Autodesk Fusion 360 part; units mm, degrees
(part 2 of 2)
  spline S109 degree 3 poles (28.856, 5.5784) (28.9294, 5.4954) (29.0682, 5.3385) (29.2744, 5.3081) (29.3716, 5.2937) knots 0 0 0 0 0.032048 0.06061 0.06061 0.06061 0.06061
  spline S110 degree 3 poles (29.3716, 5.2937) (29.4328, 5.2987) (29.5558, 5.3088) (29.6585, 5.3774) (29.71, 5.4119) knots 0 0 0 0 0.018102 0.036374 0.036374 0.036374 0.036374
  spline S111 degree 3 poles (29.71, 5.4119) (29.7609, 5.46) (29.8723, 5.5653) (29.9342, 5.706) (29.9678, 5.7825) knots 0 0 0 0 0.020804 0.045551 0.045551 0.045551 0.045551
  spline S112 degree 3 poles (29.9678, 5.7825) (29.9978, 5.8777) (30.0869, 6.1604) (30.1638, 6.4466) (30.2149, 6.6365) knots 0 0 0 0 0.029943 0.088911 0.088911 0.088911 0.088911
  spline S113 degree 3 poles (30.2149, 6.6365) (30.2924, 6.9284) (30.4207, 7.4117) (30.5964, 7.8798) (30.6661, 8.0652) knots 0 0 0 0 0.090525 0.149905 0.149905 0.149905 0.149905
  spline S114 degree 3 poles (30.6661, 8.0652) (30.7287, 8.1929) (30.8511, 8.4425) (31.066, 8.6184) (31.1709, 8.7043) knots 0 0 0 0 0.042122 0.082304 0.082304 0.082304 0.082304
  spline S115 degree 3 poles (31.1709, 8.7043) (31.2926, 8.7716) (31.5496, 8.9138) (31.8434, 8.9279) (31.9981, 8.9353) knots 0 0 0 0 0.041152 0.086904 0.086904 0.086904 0.086904
  spline S116 degree 3 poles (31.9981, 8.9353) (32.1582, 8.9226) (32.4839, 8.8969) (32.7671, 8.7336) (32.9112, 8.6506) knots 0 0 0 0 0.047533 0.09672 0.09672 0.09672 0.09672
  spline S117 degree 3 poles (32.9112, 8.6506) (33.0461, 8.544) (33.326, 8.3228) (33.4879, 8.0045) (33.5718, 7.8396) knots 0 0 0 0 0.050952 0.105714 0.105714 0.105714 0.105714
  spline S118 degree 3 poles (33.5718, 7.8396) (33.6392, 7.6526) (33.7791, 7.2639) (33.7947, 6.8508) (33.8028, 6.6365) knots 0 0 0 0 0.059254 0.123162 0.123162 0.123162 0.123162
  line L39 (31.4234, 28.6204) -> (33.6739, 27.1218)
  line L40 (33.6739, 27.1218) -> (33.6739, 25.9509)
  line L41 (33.6739, 25.9509) -> (30.709, 28.0349)
  line L42 (30.709, 28.0349) -> (27.9698, 26.1067)
  line L43 (27.9698, 26.1067) -> (27.9698, 27.3152)
  line L44 (27.9698, 27.3152) -> (29.3072, 28.1907)
  spline S119 degree 3 poles (29.3072, 28.1907) (29.4235, 28.2657) (29.6344, 28.4017) (29.8498, 28.5304) (29.9463, 28.5881) knots 0 0 0 0 0.041534 0.075271 0.075271 0.075271 0.075271
  spline S120 degree 3 poles (29.9463, 28.5881) (29.8345, 28.6632) (29.6229, 28.8052) (29.4156, 28.9534) (29.3179, 29.0232) knots 0 0 0 0 0.040409 0.076436 0.076436 0.076436 0.076436
  line L45 (29.3179, 29.0232) -> (27.9698, 29.9846)
  line L46 (27.9698, 29.9846) -> (27.9698, 31.1394)
  line L47 (27.9698, 31.1394) -> (30.6553, 29.1682)
  line L48 (30.6553, 29.1682) -> (33.6739, 31.2898)
  line L49 (33.6739, 31.2898) -> (33.6739, 30.1028)
  line L50 (33.6739, 30.1028) -> (31.9014, 28.9319)
  line L51 (31.9014, 28.9319) -> (31.4234, 28.6204)
  line L52 (25.7998, -8.5315) -> (33.6739, -8.5315)
  line L53 (33.6739, -8.5315) -> (33.6739, -9.4983)
  line L54 (33.6739, -9.4983) -> (25.7998, -9.4983)
  line L55 (25.7998, -9.4983) -> (25.7998, -8.5315)
  spline S121 degree 3 poles (33.8028, -19.0427) (33.7932, -19.3779) (33.776, -19.9835) (33.4752, -20.5065) (33.3409, -20.74) knots 0 0 0 0 0.0987 0.178335 0.178335 0.178335 0.178335
  spline S122 degree 3 poles (33.3409, -20.74) (33.1602, -20.9172) (32.7758, -21.2942) (32.2499, -21.4164) (31.9712, -21.4812) knots 0 0 0 0 0.074478 0.158426 0.158426 0.158426 0.158426
  line L56 (31.9712, -21.4812) -> (31.8208, -20.5252)
  spline S123 degree 3 poles (31.8208, -20.5252) (31.9981, -20.4901) (32.3343, -20.4235) (32.5837, -20.1898) (32.7017, -20.0794) knots 0 0 0 0 0.052976 0.100497 0.100497 0.100497 0.100497
  spline S124 degree 3 poles (32.7017, -20.0794) (32.7908, -19.9356) (32.9858, -19.621) (33.0001, -19.2497) (33.0079, -19.0481) knots 0 0 0 0 0.049907 0.109217 0.109217 0.109217 0.109217
  spline S125 degree 3 poles (33.0079, -19.0481) (33.0034, -18.8495) (32.9954, -18.496) (32.8173, -18.1927) (32.7393, -18.0598) knots 0 0 0 0 0.058395 0.103914 0.103914 0.103914 0.103914
  spline S126 degree 3 poles (32.7393, -18.0598) (32.647, -17.9659) (32.4698, -17.7856) (32.2198, -17.7531) (32.1001, -17.7376) knots 0 0 0 0 0.038273 0.073449 0.073449 0.073449 0.073449
  spline S127 degree 3 poles (32.1001, -17.7376) (31.9964, -17.75) (31.7863, -17.7751) (31.6523, -17.9392) (31.5845, -18.0222) knots 0 0 0 0 0.030125 0.060991 0.060991 0.060991 0.060991
  spline S128 degree 3 poles (31.5845, -18.0222) (31.5331, -18.1368) (31.3904, -18.4545) (31.309, -18.7936) (31.2569, -19.0105) knots 0 0 0 0 0.037609 0.104304 0.104304 0.104304 0.104304
  spline S129 degree 3 poles (31.2569, -19.0105) (31.181, -19.3132) (31.0553, -19.8147) (30.8689, -20.2966) (30.795, -20.4876) knots 0 0 0 0 0.093498 0.154885 0.154885 0.154885 0.154885
  spline S130 degree 3 poles (30.795, -20.4876) (30.7245, -20.6144) (30.5877, -20.8607) (30.3619, -21.029) (30.2525, -21.1106) knots 0 0 0 0 0.042979 0.083454 0.083454 0.083454 0.083454
  spline S131 degree 3 poles (30.2525, -21.1106) (30.1327, -21.1717) (29.8912, -21.2948) (29.6207, -21.3116) (29.4844, -21.3201) knots 0 0 0 0 0.039882 0.080371 0.080371 0.080371 0.080371
  spline S132 degree 3 poles (29.4844, -21.3201) (29.3604, -21.3132) (29.1151, -21.2997) (28.8914, -21.1983) (28.7808, -21.1482) knots 0 0 0 0 0.036909 0.072993 0.072993 0.072993 0.072993
  spline S133 degree 3 poles (28.7808, -21.1482) (28.6764, -21.0841) (28.4679, -20.9561) (28.3147, -20.7653) (28.2383, -20.6702) knots 0 0 0 0 0.036467 0.072787 0.072787 0.072787 0.072787
  spline S134 degree 3 poles (28.2383, -20.6702) (28.1837, -20.5832) (28.0633, -20.3918) (27.9958, -20.1758) (27.959, -20.0579) knots 0 0 0 0 0.030679 0.06755 0.06755 0.06755 0.06755
  spline S135 degree 3 poles (27.959, -20.0579) (27.9246, -19.9234) (27.8541, -19.6485) (27.8453, -19.3649) (27.8409, -19.22) knots 0 0 0 0 0.041509 0.084847 0.084847 0.084847 0.084847
  spline S136 degree 3 poles (27.8409, -19.22) (27.847, -19.0084) (27.8586, -18.6073) (27.9779, -18.2245) (28.0342, -18.0437) knots 0 0 0 0 0.063161 0.119704 0.119704 0.119704 0.119704
  spline S137 degree 3 poles (28.0342, -18.0437) (28.0998, -17.8884) (28.2217, -17.5995) (28.4534, -17.3891) (28.5606, -17.2918) knots 0 0 0 0 0.049846 0.092769 0.092769 0.092769 0.092769
  spline S138 degree 3 poles (28.5606, -17.2918) (28.6858, -17.2165) (28.9587, -17.0523) (29.2719, -16.9916) (29.4414, -16.9588) knots 0 0 0 0 0.04349 0.094818 0.094818 0.094818 0.094818
  line L57 (29.4414, -16.9588) -> (29.5704, -17.9041)
  spline S139 degree 3 poles (29.5704, -17.9041) (29.433, -17.9341) (29.1666, -17.9924) (28.9754, -18.1862) (28.8829, -18.28) knots 0 0 0 0 0.041191 0.079875 0.079875 0.079875 0.079875
  spline S140 degree 3 poles (28.8829, -18.28) (28.811, -18.4005) (28.6518, -18.6673) (28.6414, -18.9791) (28.6358, -19.1502) knots 0 0 0 0 0.041435 0.091767 0.091767 0.091767 0.091767
  spline S141 degree 3 poles (28.6358, -19.1502) (28.6373, -19.3447) (28.64, -19.6799) (28.7922, -19.9764) (28.856, -20.1008) knots 0 0 0 0 0.057333 0.098767 0.098767 0.098767 0.098767
  spline S142 degree 3 poles (28.856, -20.1008) (28.9294, -20.1838) (29.0682, -20.3407) (29.2744, -20.3711) (29.3716, -20.3855) knots 0 0 0 0 0.032048 0.06061 0.06061 0.06061 0.06061
  spline S143 degree 3 poles (29.3716, -20.3855) (29.4328, -20.3805) (29.5558, -20.3704) (29.6585, -20.3018) (29.71, -20.2673) knots 0 0 0 0 0.018102 0.036374 0.036374 0.036374 0.036374
  spline S144 degree 3 poles (29.71, -20.2673) (29.7609, -20.2192) (29.8723, -20.1139) (29.9342, -19.9732) (29.9678, -19.8967) knots 0 0 0 0 0.020804 0.045551 0.045551 0.045551 0.045551
  spline S145 degree 3 poles (29.9678, -19.8967) (29.9978, -19.8015) (30.0869, -19.5188) (30.1638, -19.2326) (30.2149, -19.0427) knots 0 0 0 0 0.029943 0.088911 0.088911 0.088911 0.088911
  spline S146 degree 3 poles (30.2149, -19.0427) (30.2924, -18.7508) (30.4207, -18.2675) (30.5964, -17.7994) (30.6661, -17.614) knots 0 0 0 0 0.090525 0.149905 0.149905 0.149905 0.149905
  spline S147 degree 3 poles (30.6661, -17.614) (30.7287, -17.4863) (30.8511, -17.2367) (31.066, -17.0608) (31.1709, -16.9749) knots 0 0 0 0 0.042122 0.082304 0.082304 0.082304 0.082304
  spline S148 degree 3 poles (31.1709, -16.9749) (31.2926, -16.9076) (31.5496, -16.7654) (31.8434, -16.7513) (31.9981, -16.7439) knots 0 0 0 0 0.041152 0.086904 0.086904 0.086904 0.086904
  spline S149 degree 3 poles (31.9981, -16.7439) (32.1582, -16.7566) (32.4839, -16.7823) (32.7671, -16.9456) (32.9112, -17.0286) knots 0 0 0 0 0.047533 0.09672 0.09672 0.09672 0.09672
  spline S150 degree 3 poles (32.9112, -17.0286) (33.0461, -17.1352) (33.326, -17.3564) (33.4879, -17.6747) (33.5718, -17.8396) knots 0 0 0 0 0.050952 0.105714 0.105714 0.105714 0.105714
  spline S151 degree 3 poles (33.5718, -17.8396) (33.6392, -18.0266) (33.7791, -18.4153) (33.7947, -18.8284) (33.8028, -19.0427) knots 0 0 0 0 0.059253 0.123162 0.123162 0.123162 0.123162
  line L58 (-53.5, 35.5) -> (-50, 35.5)
  line L59 (-45.3, 35.5) -> (-50, 35.5)
  line L60 (-45.3, 35.5) -> (-45.3, 41)
  line L61 (-50, 41) -> (-45.3, 41)
  line L62 (-50.5, 41) -> (-50, 41)
  spline S152 degree 3 poles (-53.5, 38) (-53.5, 38.0045) (-53.5, 38.009) (-53.4999, 38.0252) (-53.4998, 38.0369) (-53.4993, 38.0696) (-53.4987, 38.0904) (-53.4952, 38.1851) (-53.4897, 38.2602) (-53.4713, 38.4231) (-53.4585, 38.502) (-53.4129, 38.7374) (-53.3666, 38.895) (-53.1898, 39.3824) (-52.9511, 39.8247) (-52.2876, 40.4301) (-52.0001, 40.6252) (-51.2823, 40.9238) (-50.891, 41) (-50.5, 41) knots 2.040381 2.040381 2.040381 2.040381 2.042337 2.042337 2.047449 2.047449 2.056776 2.056776 2.090755 2.090755 2.128283 2.128283 2.220621 2.220621 2.480076 2.480076 2.621897 2.621897 2.772747 2.772747 2.772747 2.772747
  line L63 (-53.5, 38) -> (-53.5, 35.5)
  line L64 (-50, -35.5) -> (-53.5, -35.5)
  line L65 (-53.5, -35.5) -> (-53.5, -38)
  spline S153 degree 3 poles (-50.5, -41) (-50.7331, -41) (-50.9678, -40.9728) (-51.6012, -40.8211) (-51.9827, -40.6426) (-52.9395, -39.9115) (-53.2354, -39.3177) (-53.3988, -38.7785) (-53.4261, -38.6718) (-53.4608, -38.4885) (-53.4736, -38.4073) (-53.4908, -38.246) (-53.4957, -38.175) (-53.4988, -38.0855) (-53.4993, -38.0661) (-53.4998, -38.035) (-53.4999, -38.0236) (-53.5, -38.008) (-53.5, -38.004) (-53.5, -38) knots 1.485719 1.485719 1.485719 1.485719 1.554373 1.554373 1.673928 1.673928 1.89203 1.89203 1.936507 1.936507 1.963659 1.963659 1.985978 1.985978 1.99201 1.99201 1.995484 1.995484 1.996683 1.996683 1.996683 1.996683
  line L66 (-45.3, -41) -> (-50.5, -41)
  line L67 (-45.3, -41) -> (-45.3, -35.5)
  line L68 (-50, -35.5) -> (-45.3, -35.5)
  line L69 (-8, -41) -> (-8, -4)
  line L70 (-8, -4) -> (9, -4)
  line L71 (9, -4) -> (9, 41)
  line L72 (-53.5, -35.5) -> (-53.5, 35.5)
  line L73 (-41.1, 29.5) -> (-41.1, 35.5)
  line L74 (-53.5, 29.5) -> (-41.1, 29.5)
  line L75 (-53.5, -29.5) -> (-41.1, -29.5)
  line L76 (-41.1, -29.5) -> (-41.1, -35.5)
  line L77 (-53.5, -35.5) -> (-53.5, -29.5)
  line L78 (-53.5, 35.5) -> (-53.5, 29.5)
  line L79 (-41.1, 32.5) -> (-53.5, 32.5) construction
  line L80 (-41.1, 35) -> (-53.5, 35)
  line L81 (-53.5, 35) -> (-53.5, 30)
  line L82 (-53.5, 30) -> (-41.1, 30)
  line L83 (-41.1, 30) -> (-41.1, 35)
  line L84 (0, 0) -> (-53.5, 0) construction
  line L85 (-41.1, -35) -> (-53.5, -35)
  line L86 (-53.5, -30) -> (-41.1, -30)
  dimension "d202" = 1
  dimension "d203" = 1
  dimension "d204" = 1
  dimension "d211" = 5
  constraint coincident L13 L69.start
  constraint perpendicular L13 L69
  constraint perpendicular L21 L70
  constraint coincident L15 L71.end
  constraint perpendicular L15 L71
  constraint coincident L64.end L65.start
  constraint coincident L58.start L63.end
  constraint midpoint L73 L79.start
  constraint midpoint L78 L79.end
  constraint horizontal L80
  constraint vertical L81
  constraint horizontal L82
  constraint vertical L83
  constraint midpoint L79.start L83
  constraint midpoint L79.end L81
  constraint coincident L84.start origin
  constraint midpoint L72 L84.end
  constraint symmetric L80.start L84 L85.start
  constraint symmetric L80.end L84 L85.end
  constraint symmetric L81.end L84 L86.start
  constraint symmetric L82.end L84 L86.end
  measures "d69" distance of S38.end
  measures "d202" distance of L21 L69
  measures "d203" distance of L20 L70
  measures "d204" distance of L19 L71
  measures "d211" distance of L80.start L82.end
extrude "Extrude mounts" add sketch "Bottom (2)" against normal blind 10.4 separate body contours L72 L73 L78 L80 L81 L82 L83 | L72 L76 L77 L85 L86 makes body 3 at (49.3667, -30, 41.5333) makes body 4 at (49.3667, 30, 41.5333) in component "Moving Lid"
extrude "Extrude thickness" add sketch "Bottom (2)" along normal blind 2.6 separate body contours L0 L1 L2 L3 L15 L60 L71 | L0 L58 L59 L60 L61 L62 S152 L63 | L1 L58 L59 L72 L73 L78 L80 | L2 L3 L9 L10 L69 L70 L71 L72 L73 L74 L75 L76 L83 | L72 L73 L78 L80 L81 L82 L83 | L72 L73 L74 L78 L82 | L9 L10 L11 L12 L13 L67 L69 | L72 L75 L76 L77 L86 | L12 L64 L65 S153 L66 L67 L68 | L11 L64 L68 L72 L76 L77 L85 | L72 L76 L77 L85 L86 makes body 5 in component "Moving Lid"
chamfer "Chamfer upper edge" distance 1.2 angle 55 5 edges at (20.75, -41, 47.6) (52.8428, -39.8742, 47.6) (53.5, 0, 47.6) (52.8062, 39.9199, 47.6) (29.25, 41, 47.6) measured on face at (38.3333, 1.3333, 47.6) measured on face at (38.3333, 1.3333, 47.6) measured on face at (38.3333, 1.3333, 47.6) measured on face at (38.3333, 1.3333, 47.6) measured on face at (38.3333, 1.3333, 47.6) on bodies 5 in component "Moving Lid"
chamfer "Chamfer gap edge" distance 2.6 angle 30 2 edges at (-9, -18.5, 45) (8, 22.5, 45) measured on face at (-9, -23.6667, 45.8667) measured on face at (8, 26.3333, 45.8667) on bodies 5 in component "Moving Lid"
sketch "Mount holes" plane through (0, -35, 0) normal (0, -1, 0) x (1, 0, 0) in component "Moving Lid"
  line L0 (53.5, 45) -> (41.1, 45)
  line L1 (41.1, 45) -> (41.1, 34.6)
  line L2 (41.1, 34.6) -> (53.5, 34.6)
  line L3 (53.5, 34.6) -> (53.5, 45)
  circle A0 centre (47.3, 38.8) radius 1.5
  circle A1 centre (47.3, 38.8) radius 2.25
  arc A2 (47.3, 32.6) -> (53.5, 38.8) centre (47.3, 38.8) ccw construction
  line L4 (47.3, 38.8) -> (53.5, 38.8) construction
  line L5 (47.3, 38.8) -> (47.3, 34.6) construction
  line L6 (41.1, 45) -> (53.5, 45)
  line L7 (53.5, 45) -> (53.5, 39.6)
  line L8 (48.5, 34.6) -> (46.1, 34.6)
  line L9 (41.1, 39.6) -> (41.1, 45)
  arc A3 (41.1, 39.6) -> (46.1, 34.6) centre (46.1, 39.6) ccw
  arc A4 (48.5, 34.6) -> (53.5, 39.6) centre (48.5, 39.6) ccw
  dimension "d214" = 0.75
  dimension "d215" = 5
  constraint coincident L3 A2.end
  constraint coincident A0.centre A1.centre
  constraint perpendicular L3 L4
  constraint midpoint L2 L5.end
  constraint coincident A2.end L4.end
  constraint horizontal L6
  constraint vertical L7
  constraint horizontal L8
  constraint vertical L9
  constraint coincident L0.end L1.start
  constraint tangent L9 A3
  constraint tangent L8 A3
  constraint tangent L8 A4
  constraint tangent L7 A4
  constraint equal A3 A4
  measures "d215" radius of A3
extrude "Cut mount holes" cut sketch "Mount holes" against normal up to surface (70 mm away) contours L2 L3 A4 | L1 L2 A3 | A0 | A1 bodies 3 4 in component "Moving Lid"
extrude "Extrude22" add 1 faces at (50.6667, 22.4167, 2.4) along direction (0, 0, 1) blind 12 on bodies 1 bodies 1 in component "Box Base"
ref_plane "WorkPlane2" through (0, -19.5, 23.7) normal (0, 1, 0) x (-1, 0, 0) in component "Box Base"
sketch "Motor mount" plane through (0, -19.5, 0) normal (0, 1, 0) x (1, 0, 0) in component "Box Base"
  line L0 (50, -3) -> (44.6, -3)
  line L1 (44.6, -3) -> (44.6, -16)
  line L2 (44.6, -16) -> (50, -16)
  line L3 (50, -16) -> (50, -3)
  line L4 (47.3, -3) -> (47.3, -9.3) construction
  circle A0 centre (47.3, -9.3) radius 1.25
  line L5 (44.6, -3) -> (21.4, -3) construction
  line L6 (21.4, -3) -> (16, -3)
  line L7 (16, -3) -> (16, -16)
  line L8 (16, -16) -> (21.4, -16)
  line L9 (21.4, -16) -> (21.4, -3)
  line L10 (18.7, -3) -> (18.7, -9.3) construction
  circle A1 centre (18.7, -9.3) radius 1.1
  dimension "d228" = 5.4
  dimension "d229" = 13
  dimension "d235" = 6.3
  dimension "d236" = 2.5
  dimension "d237" = 23.2
  dimension "d238" = 5.4
  dimension "d239" = 13
  dimension "d240" = 6.3
  dimension "d241" = 2.2
  constraint horizontal L0
  constraint vertical L1
  constraint horizontal L2
  constraint vertical L3
  constraint midpoint L0 L4.start
  constraint perpendicular L0 L4
  constraint coincident L4.end A0.centre
  constraint perpendicular L1 L5
  constraint horizontal L6
  constraint vertical L7
  constraint horizontal L8
  constraint vertical L9
  constraint midpoint L6 L10.start
  constraint perpendicular L6 L10
  constraint coincident L10.end A1.centre
  measures "d228" distance of L0.start L0.end
  measures "d229" distance of L0.start L2.end
  measures "d235" distance of L4.start L4.end
  measures "d236" diameter of A0
  measures "d237" distance of L0.end L5.end
  measures "d238" distance of L5.end L6.end
  measures "d239" distance of L5.end L8.end
  measures "d240" distance of L10.start L10.end
  measures "d241" diameter of A1
extrude "Extrude25" add sketch "Motor mount" along normal blind 8.5 bodies 1 makes body 6 at (21.4, -16.6667, 11.6667) in component "Box Base"
extrude "Extrude27" add 1 faces at (19.6, -16.6667, 3) along direction (0, 0, -1) blind 2.4 on bodies 6 bodies 1 6 in component "Box Base"
fillet "Fillet4" radius 4 1 edges at (16, -15.25, 2.4) on bodies 1 in component "Box Base"
component "Box Base" placed x (1, 0, 0) y (0, 1, 0) z (0, 0, 1) at (0, 0, 0)
component "Fixed Lid" placed x (1, 0, 0) y (0, 1, 0) z (0, 0, 1) at (0, 0, 0)
component "Moving Lid" placed x (1, 0, 0) y (0, 1, 0) z (0, 0, 1) at (0, 0, 0)
equation "BoxBaseInternalWidth = 75 mm"
equation "BoxBaseInternalLength = 100 mm"
equation "BoxBaseWallThickness = 3.5 mm"
equation "BoxBaseRoundedCornerRadius = 3 mm"
equation "d5 = BoxBaseInternalLength"
equation "d6 = BoxBaseInternalWidth"
equation "d7 = BoxBaseInternalWidth + BoxBaseWallThickness + BoxBaseWallThickness"
equation "d8 = BoxBaseInternalLength + BoxBaseWallThickness + BoxBaseWallThickness"
equation "d9 = BoxBaseRoundedCornerRadius"
equation "BoxBaseHeight = 45 mm"
equation "d11 = BoxBaseHeight"
equation "BoxBaseBottomThickness = 2.4 mm"
equation "d14 = BoxBaseBottomThickness"
equation "BoxBaseBottomEdgeChamfer = 2 mm"
equation "d17 = BoxBaseBottomEdgeChamfer"
equation "FixedLidWidth = 40 mm"
equation "d19 = FixedLidWidth"
equation "BoxBaseFixedLidMountWidth = 9 mm"
equation "d28 = BoxBaseFixedLidMountWidth - BoxBaseWallThickness"
equation "d31 = d28"
equation "d32 = d29"
equation "BoxBaseFixedLidScrewHoleDiameter = 3 mm"
equation "d37 = d36"
equation "d38 = BoxBaseFixedLidScrewHoleDiameter"
equation "d39 = BoxBaseFixedLidScrewHoleDiameter"
equation "BoxBaseFixedLidScrewHoleDepth = 15 mm"
equation "d41 = -BoxBaseFixedLidScrewHoleDepth"
equation "BoxBaseFixedLidScrewHoleChamfter = 1 mm"
equation "d44 = BoxBaseFixedLidScrewHoleChamfter"
equation "BoxBaseBoardWidth = 26.5 mm"
equation "BoxBaseBoardLength = 0.01 mm"
equation "BoxBaseBoardWallSupportHeight = 0.01 mm"
equation "BoxBaseBoardWallSupportThickness = 0.01 mm"
equation "BoxBaseBoardBottomSupportHeight = 0.01 mm"
equation "d50 = BoxBaseBoardLength"
equation "d51 = BoxBaseBoardWidth"
equation "d52 = BoxBaseBoardWallSupportThickness"
equation "d53 = BoxBaseBoardWallSupportThickness"
equation "d54 = BoxBaseBoardWallSupportHeight"
equation "d56 = BoxBaseBoardBottomSupportWidth"
equation "d57 = BoxBaseBoardBottomSupportHeight"
equation "BoxBaseBoardUsbHoleWidth = 11 mm"
equation "BoxBaseBoardUsbHoleHeight = 18 mm"
equation "BoxBaseBoardUsbCableWidth = 15 mm"
equation "BoxBaseBoardUsbCableHeight = 22 mm"
equation "d69 = BoxBaseBoardUsbHoleWidth"
equation "d70 = BoxBaseBoardUsbHoleHeight"
equation "d71 = BoxBaseBoardUsbCableWidth"
equation "d72 = BoxBaseBoardUsbCableHeight"
equation "d74 = -( BoxBaseWallThickness - 1 mm )"
equation "d76 = BoxBaseBottomEdgeChamfer"
equation "BoxBaseBoardBottomSupportWidth = 0.01 mm"
equation "BoxBaseShaftScrewHoleDiameter = 3 mm"
equation "BoxBaseShaftScrewHeadHoleDiameter = 6.4 mm"
equation "BoxBaseShaftScrewHeadHoleDepth = 3.5 mm"
equation "d99 = BoxBaseShaftScrewHoleDiameter"
equation "d100 = BoxBaseShaftScrewHeadHoleDiameter"
equation "d101 = BoxBaseShaftScrewHeadHoleDiameter + BoxBaseShaftScrewHoleWallThickness + BoxBaseShaftScrewHoleWallThickness"
equation "BoxBaseShaftScrewHoleWallThickness = 3 mm"
equation "d103 = d101 / 2"
equation "d104 = d103"
equation "d110 = -BoxBaseShaftScrewHeadHoleDepth"
equation "d112 = -BoxBaseShaftScrewHeadHoleDepth"
equation "OpenLidMountWidth = 5 mm"
equation "d115 = OpenLidMountWidth + 1 mm"
equation "d123 = d104 + 2 mm"
equation "d124 = d123"
equation "d128 = -d101"
equation "FixedLidScrewHoleDiameter = BoxBaseFixedLidScrewHoleDiameter + 0.8 mm"
equation "d132 = FixedLidScrewHoleDiameter"
equation "d133 = FixedLidScrewHoleDiameter"
equation "d134 = FixedLidScrewHoleDiameter"
equation "d135 = FixedLidScrewHoleDiameter"
equation "LidThickness = 2.6 mm"
equation "FixedLidSwitchHoleDiameter = 6.7 mm"
equation "d138 = FixedLidSwitchHoleDiameter"
equation "FixedLidSwitchHoleDistance = 11.5 mm"
equation "d140 = FixedLidSwitchHoleDistance"
equation "FixedLidExtensionLength = 17 mm"
equation "d143 = FixedLidExtensionLength"
equation "FixedLidArmHoleWidth = 10 mm"
equation "d145 = FixedLidArmHoleWidth / 2"
equation "d146 = LidThickness"
equation "LidUpperEdgeChamfer = 1.2 mm"
equation "d149 = LidUpperEdgeChamfer"
equation "FixedLidSensorHoleDiameter = 6.2 mm"
equation "d152 = FixedLidSensorHoleDiameter"
equation "FixedLidSensorLength = 16 mm"
equation "FixedLidSensorWidth = 21 mm"
equation "FixedLidSensorSupportWallThickness = 2 mm"
equation "d156 = FixedLidSensorLength"
equation "d157 = FixedLidSensorWidth"
equation "d158 = -FixedLidSensorSupportWallThickness"
equation "FixedLidSensorHoleDistanceFromEdge = 5 mm"
equation "d160 = FixedLidSensorHoleDistanceFromEdge"
equation "FixedLidSensorSupportWallHeight = 4 mm"
equation "d162 = FixedLidSensorSupportWallHeight"
equation "MotorMountWidth = 5.4 mm"
equation "MotorMountHeight = 13 mm"
equation "MotorMountDepth = 8.5 mm"
equation "MotorMountHoleDiameter = 2.2 mm"
equation "MotorMountDistance = 23.2 mm"
equation "FixedLidMotorMountDistanceFromCenter = 15 mm"
equation "d170 = FixedLidMotorMountDistanceFromCenter"
equation "d171 = MotorMountDepth"
equation "d172 = MotorMountWidth"
equation "d173 = d170"
equation "d174 = d171"
equation "d175 = d172"
equation "d176 = MotorMountDistance"
equation "d177 = MotorMountHeight"
equation "d179 = MotorMountHoleDiameter"
equation "d180 = d179"
equation "MotorMountHoleDistanceFromEdge = 6.3 mm"
equation "d182 = MotorMountHoleDistanceFromEdge"
equation "d183 = d182"
equation "FixedLidSensorMountWidth = 4.3 mm"
equation "FixedLidSensorMountHeight = 1.6 mm"
equation "FixedLidSensorMountScrewHoleDiameter = 2.5 mm"
equation "d192 = MotorMountWidth"
equation "d193 = MotorMountWidth"
equation "d194 = MotorMountWidth"
equation "d195 = MotorMountWidth"
equation "d196 = FixedLidSensorMountScrewHoleDiameter"
equation "d197 = FixedLidSensorMountScrewHoleDiameter"
equation "d198 = FixedLidSensorMountHeight"
equation "OpenLidGap = 1.0 mm"
equation "OpenLidGapBottomChamfer = LidThickness"
equation "d202 = OpenLidGap"
equation "d203 = OpenLidGap"
equation "d204 = OpenLidGap"
equation "d205 = LidThickness"
equation "d207 = LidUpperEdgeChamfer"
equation "d209 = OpenLidGapBottomChamfer"
equation "d211 = OpenLidMountWidth"
equation "d212 = -( d101 - 2 mm )"
equation "d219 = BoxBaseBoardUsbHoleHeightBottom"
equation "BaseMotorMountDistanceFromWall = 18 mm"
equation "d227 = BaseMotorMountDistanceFromWall"
equation "d228 = MotorMountWidth"
equation "d229 = MotorMountHeight"
equation "d235 = MotorMountHoleDistanceFromEdge"
equation "d236 = FixedLidSensorMountScrewHoleDiameter"
equation "d237 = MotorMountDistance"
equation "d238 = MotorMountWidth"
equation "d239 = MotorMountHeight"
equation "d240 = MotorMountHoleDistanceFromEdge"
equation "d241 = MotorMountHoleDiameter"
equation "d242 = MotorMountDepth"
equation "BoxBaseBoardUsbHoleHeightBottom = 12 mm"
equation "d249 = BoxBaseBottomThickness"
named bodies: "Base", "Fixed Lid"
